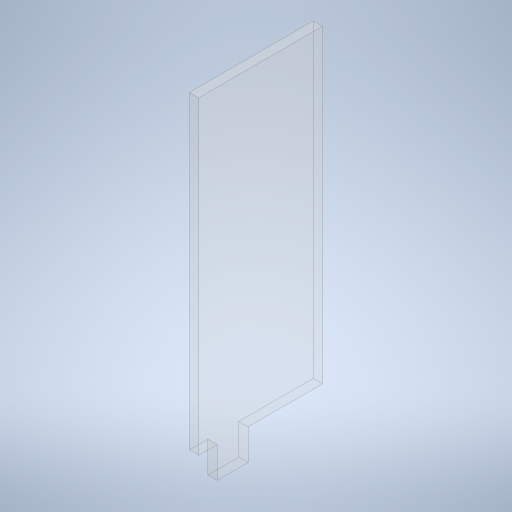
# Autodesk Inventor part: Arcylic_Panel_Base_20mm_P1
Saved by Autodesk Inventor 2023 (Build 270158000, 158)
## iProperties
Created: 2022-09-10
Part Number: Arcylic_Panel_Base_20mm_P1
Material: Generic
Document SubType Name: Modeling
Designer: Desmond
Density: 1 g/cm^3
Appearance: Polycarbonate - Clear
Author: Desmond
Autodesk Inventor part; units mm, degrees
ref_plane "YZ Plane" through (0, 0, 0) normal (1, 0, 0) x (0, 1, 0)
ref_plane "XZ Plane" through (0, 0, 0) normal (0, 1, 0) x (-1, 0, 0)
ref_plane "XY Plane" through (0, 0, 0) normal (0, 0, 1) x (1, 0, 0)
sketch "Sketch1" plane through (0, 0, 0) normal (0, 1, 0) x (-1, 0, 0)
  line L0 (0.7432, 9.5847) -> (-0.7568, 9.5847)
  line L1 (-0.7568, 9.5847) -> (-0.7568, -10.4153)
  line L2 (-0.7568, -10.4153) -> (0.7432, -10.4153)
  line L3 (0.7432, -10.4153) -> (0.7432, 9.5847)
  point P0 (0, 0)
  dimension "d0" = 20
  dimension "d1" = 1.5
  constraints: 8 end point, 2 parallel, 1 horizontal, 1 perpendicular
  measures "d0" distance of L2.end L0.start
  measures "d1" distance of L0.start L0.end
extrude "Extrusion1" add sketch "Sketch1" along normal blind 50
sketch "Sketch3" plane through (0, 0, 0) normal (0, -1, 0) x (1, 0, 0)
  line L0 (-0.7432, -10.4153) -> (-0.7432, 9.5847) projected
  line L1 (0.7568, 9.5847) -> (0.7568, -10.4153) projected
  line L2 (-0.7432, 6.59) -> (0.7568, 6.59)
  line L3 (0.7568, 6.59) -> (0.7568, 1.59)
  line L4 (0.7568, 1.59) -> (-0.7432, 1.59)
  line L5 (-0.7432, 1.59) -> (-0.7432, 6.59)
  line L6 (-0.7432, -2.11) -> (0.7568, -2.11)
  line L7 (0.7568, -2.11) -> (0.7568, -7.11)
  line L8 (0.7568, -7.11) -> (-0.7432, -7.11)
  line L9 (-0.7432, -7.11) -> (-0.7432, -2.11)
  point P0 (0, 0)
  point P1 (-0.7432, 1.59)
  point P2 (0.7568, 6.59)
  dimension "d4" = 5
  dimension "d5" = 5
  constraints: 16 end point, 4 parallel, 4 point on line, 2 horizontal, 2 perpendicular
  measures "d4" distance of L2.end L3.end
  measures "d5" distance of L6.end L7.end
extrude "Extrusion2" add sketch "Sketch3" along normal blind 5 contours L0 L2 L1 L4
body "Solid1"
